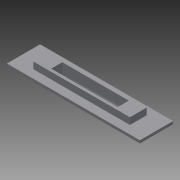
# Autodesk Inventor part: Part1
Saved by Autodesk Inventor 2015 (Build 190159000, 159)
## iProperties
Created: 2016-09-18
Part Number: Part1
Material: Generic
Document SubType Name: Modeling
Designer: Administrator
Density: 1 g/cm^3
Appearance: Default
Author: Administrator
Autodesk Inventor part; units mm, degrees
ref_plane "YZ Plane" through (0, 0, 0) normal (1, 0, 0) x (0, 1, 0)
ref_plane "XZ Plane" through (0, 0, 0) normal (0, 1, 0) x (-1, 0, 0)
ref_plane "XY Plane" through (0, 0, 0) normal (0, 0, 1) x (1, 0, 0)
sketch "Sketch1" plane through (0, 0, 0) normal (0, 0, 1) x (1, 0, 0)
  line L0 (-30, 7.5) -> (30, 7.5)
  line L1 (30, 7.5) -> (30, -7.5)
  line L2 (30, -7.5) -> (-30, -7.5)
  line L3 (-30, -7.5) -> (-30, 7.5)
  line L4 (-42, 0) -> (42, 0) projected
  line L5 (0, -10.5) -> (0, 10.5) projected
  line L6 (-15, 2.5) -> (15, 2.5)
  line L7 (15, 2.5) -> (15, -2.5)
  line L8 (15, -2.5) -> (-15, -2.5)
  line L9 (-15, -2.5) -> (-15, 2.5)
  point P0 (0, 0)
  dimension "d0" = 30
  dimension "d1" = 5
  dimension "d2" = 60
  dimension "d3" = 15
  constraints: 16 end point, 4 parallel, 4 symmetric about line, 2 horizontal, 2 perpendicular
  measures "d0" distance of L6.start L6.end
  measures "d1" distance of L6.end L7.end
  measures "d2" distance of L0.start L0.end
  measures "d3" distance of L0.end L1.end
extrude "Extrusion1" add sketch "Sketch1" along normal blind 1.2 contours L0 L5 L6 L9 L4 L3 | L0 L1 L4 L7 L6 L5 | L4 L9 L8 L5 L2 L3 | L1 L2 L5 L8 L7 L4
sketch "Sketch2" plane through (0, 0, 1.2) normal (0, 0, 1) x (1, 0, 0)
  line L0 (0, -10.5) -> (0, 10.5) projected
  line L1 (-42, 0) -> (42, 0) projected
  line L2 (-21.75, 3.75) -> (21.75, 3.75)
  line L3 (21.75, 3.75) -> (21.75, -3.75)
  line L4 (21.75, -3.75) -> (-21.75, -3.75)
  line L5 (-21.75, -3.75) -> (-21.75, 3.75)
  line L6 (-15, -2.5) -> (-15, 2.5) projected
  line L7 (-15, 2.5) -> (15, 2.5) projected
  line L8 (15, -2.5) -> (-15, -2.5) projected
  line L9 (15, 2.5) -> (15, -2.5) projected
  point P0 (0, 0)
  dimension "d6" = 43.5
  dimension "d7" = 7.5
  constraints: 8 end point, 2 parallel, 2 symmetric about line, 1 horizontal, 1 perpendicular
  measures "d6" distance of L3.end L4.end
  measures "d7" distance of L4.end L2.start
extrude "Extrusion2" add sketch "Sketch2" along normal blind 3 contours L4 L5 L1 L6 L8 L0 | L0 L8 L9 L1 L3 L4 | L1 L9 L7 L0 L2 L3 | L5 L2 L0 L7 L6 L1
body "Solid1"
